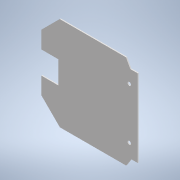
# Autodesk Inventor part: PCB
Saved by Autodesk Inventor 2020 (Build 240168000, 168)
## iProperties
Created: 2020-04-22
Part Number: PCB
Material: Genérico
Document SubType Name: Modeling
Designer: gi-se
Density: 1 g/cm^3
Appearance: Padrão
Author: gi-se
Autodesk Inventor part; units mm, degrees
ref_plane "YZ Plane" through (0, 0, 0) normal (1, 0, 0) x (0, 1, 0)
ref_plane "XZ Plane" through (0, 0, 0) normal (0, 1, 0) x (-1, 0, 0)
ref_plane "XY Plane" through (0, 0, 0) normal (0, 0, 1) x (1, 0, 0)
sketch "Esboço1" plane through (0, 0, 0) normal (0, 0, 1) x (1, 0, 0)
  line L0 (88, 16) -> (56, 16) projected
  line L1 (88, -64) -> (56, -64) projected
  line L2 (116, -64.0154) -> (116, 11.5655)
  line L3 (-8, -88.1) -> (-8, -95.9) projected
  line L4 (38.5088, -95.9) -> (-8, -95.9) projected
  line L5 (38.5088, -95.9) -> (38.5088, -88.1) projected
  line L6 (38.5088, 47.9) -> (38.5088, 40.1) projected
  line L7 (38.5088, 47.9) -> (-8, 47.9) projected
  line L8 (-8, 40.1) -> (-8, 47.9) projected
  line L9 (99.6, 47.9) -> (99.6, 40.1)
  line L10 (-11.6, -95.9) -> (-11.6, -88.1)
  line L11 (-20, -64) -> (6.1, -90.1)
  line L12 (-20, -64) -> (16.911, -64) construction
  line L13 (-20.13, 16) -> (5.97, 42.1)
  line L14 (-20.13, 16) -> (16.781, 16) construction
  line L15 (99.3981, 42.1) -> (5.97, 42.1)
  line L16 (6.1, -90.1) -> (99.6, -90.1)
  line L17 (116, -64.0154) -> (99.6, -90.1)
  line L18 (99.3981, 42.1) -> (116, 11.5655)
  line L19 (4, -8) -> (-20.13, -8)
  line L20 (-20, -40) -> (4, -40)
  line L21 (4, -40) -> (4, -8)
  line L22 (-20.13, 16) -> (-20.13, -8)
  line L23 (-20, -40) -> (-20, -64)
  spline S0 degree 3 poles (105.3201, 14.0044) (105.3235, 14.0021) (105.3286, 13.9988) (105.3629, 13.9756) (105.3885, 13.9579) (105.4461, 13.9157) (105.482, 13.8884) (105.5584, 13.8259) (105.5988, 13.7906) (105.6725, 13.722) (105.7105, 13.6842) (105.7783, 13.6124) (105.8082, 13.5785) (105.8543, 13.5241) (105.8738, 13.4998) (105.8993, 13.4673) (105.903, 13.4624) (105.9055, 13.4591) knots -0.241565 -0.241565 -0.241565 -0.241565 -0.226467 -0.226467 -0.211369 -0.211369 -0.196271 -0.196271 -0.181173 -0.181173 -0.166076 -0.166076 -0.150978 -0.150978 -0.13588 -0.13588 -0.120782 -0.120782 -0.120782 -0.120782 projected
  circle A0 centre (104, 12) radius 2.4
  spline S1 degree 3 poles (105.3201, -57.9956) (105.3235, -57.9979) (105.3286, -58.0012) (105.3629, -58.0244) (105.3885, -58.0421) (105.4461, -58.0843) (105.482, -58.1116) (105.5584, -58.1741) (105.5988, -58.2094) (105.6725, -58.278) (105.7105, -58.3158) (105.7783, -58.3876) (105.8082, -58.4215) (105.8543, -58.4759) (105.8738, -58.5002) (105.8993, -58.5327) (105.903, -58.5376) (105.9055, -58.5409) knots -0.241565 -0.241565 -0.241565 -0.241565 -0.226467 -0.226467 -0.211369 -0.211369 -0.196271 -0.196271 -0.181173 -0.181173 -0.166076 -0.166076 -0.150978 -0.150978 -0.13588 -0.13588 -0.120782 -0.120782 -0.120782 -0.120782 projected
  circle A1 centre (104, -60) radius 2.4
  line L24 (64, 40.1) -> (96, 40.1) projected
  line L25 (-20.13, -23.115) -> (-20.13, 8) projected
  line L26 (56, -24) -> (88, -24) projected
  line L27 (115.1988, -78.8) -> (116, -78.8) projected
  line L28 (115.1988, 30.8) -> (116, 30.8) projected
  line L29 (116, 30.8) -> (105.542, 30.8)
  line L30 (116, -78.8) -> (106.7046, -78.8)
  line L31 (116, -78.8) -> (116, -64.0154)
  line L32 (116, 11.5655) -> (116, 30.8)
  point P0 (105.4155, 13.9381)
  point P1 (105.8855, 13.4849)
  point P2 (105.4436, -58.0827)
  point P3 (105.8098, -58.4238)
  dimension "d20" = 45
  dimension "d21" = 45
  dimension "d22" = 2
  dimension "d24" = 0
  dimension "d25" = 24
  dimension "d26" = 16
  constraints: 40 end point, 5 horizontal, 4 parallel, 3 point on line, 2 centre point, 2 collinear, 2 equal length, 2 vertical, 4 other
  measures "d20" angle of L11 L12
  measures "d21" angle of L14 L13
  measures "d22" distance between parallel lines of L15 L24
  measures "d24" distance between parallel lines of L25 L22
  measures "d25" distance from line of L19 L13.start
  measures "d26" distance between parallel lines of L19 L26
extrude "Extrusão1" add sketch "Esboço1" along normal blind 1.5
